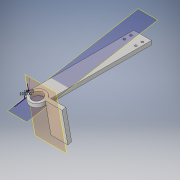
# Autodesk Inventor part: WheelIntakeMotorMount2.0
Saved by Autodesk Inventor 2017 (Build 210142000, 142)
## iProperties
Created: 2017-11-18
Part Number: WheelIntakeMotorMount2.0
Material: Generic
Document SubType Name: Modeling
Designer: User
Density: 1 g/cm^3
Appearance: Default
Author: User
Autodesk Inventor part; units mm, degrees
ref_plane "YZ Plane" through (0, 0, 0) normal (1, 0, 0) x (0, 1, 0)
ref_plane "XZ Plane" through (0, 0, 0) normal (0, 1, 0) x (-1, 0, 0)
ref_plane "XY Plane" through (0, 0, 0) normal (0, 0, 1) x (1, 0, 0)
sketch "Sketch1" plane through (0, 0, 0) normal (1, 0, 0) x (0, 1, 0)
  line L0 (0, 0) -> (21.59, 0)
  line L1 (21.59, 0) -> (21.59, -127)
  line L2 (21.59, -127) -> (0, -127)
  line L3 (0, -127) -> (0, 0)
  dimension "d0" = 21.59
  dimension "d1" = 127
  constraints: 8 end point, 2 parallel, 1 horizontal, 1 perpendicular
  measures "d0" distance of L1.end L2.end
  measures "d1" distance of L0.end L1.end
extrude "Extrusion1" add sketch "Sketch1" along normal blind 4.7625
sketch "Sketch2" plane through (0, 21.59, 0) normal (0, 1, 0) x (1, 0, 0)
  line L0 (0, 0) -> (-3.2071, -18.1884)
  line L1 (0, 0) -> (18.469, 0) construction
  line L2 (0, 0) -> (13.0579, -2.3025)
  line L3 (0, 0) -> (13.2594, 0) construction
  dimension "d4" = 100
  dimension "d24" = 10
  constraints: 8 end point, 2 equal length, 2 horizontal
  measures "d4" angle of L0 L1
  measures "d24" angle of L2 L3
ref_plane "Work Plane1" through (0, 21.59, 0) normal (-0.9848078, 0, -0.1736482) x (-0.1736482, 0, 0.9848078)
sketch "Sketch3" plane through (0, 21.59, 0) normal (-0.9848078, 0, -0.1736482) x (-0.1736482, 0, 0.9848078)
  line L0 (-0.827, 0) -> (-0.827, -21.59) projected
  line L1 (-0.827, -21.59) -> (-125.8976, -21.59) projected
  line L2 (-125.8976, -21.59) -> (-125.8976, 0) projected
  line L3 (-125.8976, 0) -> (-0.827, 0) projected
  line L4 (0, -21.59) -> (0, 0) projected
  line L5 (0, -21.59) -> (-0.827, -21.59) projected
  line L6 (-0.827, 0) -> (-0.827, -21.59) projected
  line L7 (0, 0) -> (-0.827, 0) projected
  line L8 (0, -21.59) -> (0, 0) projected
  circle A0 centre (0, -10.795) radius 9.525
  dimension "d5" = 19.05
  dimension "d6" = 21.59
  dimension "d7" = 10.795
  constraints: 1 centre point, 1 midpoint
  measures "d5" diameter of A0
  measures "d6" distance of L4.start L4.end
  measures "d7" distance from line of L7 A0.centre
extrude "Extrusion2" add sketch "Sketch3" against normal blind 4.7625 contours A0 L4 L0 | L0 A0 | A0 L4
sketch "Sketch5" plane through (4.6901, 10.795, 0.827) normal (0.9848078, 0, 0.1736482) x (0.1736482, 0, -0.9848078)
  circle A0 centre (0, 0) radius 9.525 projected
  point P0 (0, -10.795)
hole "Hole2" at (4.6901, 10.795, 0.827) direction (-0.9848078, 0, -0.1736482) diameter 12.954 end through all
ref_plane "Work Plane3" through (0, 0, 0) normal (-0.1736482, 0, 0.9848078) x (0, 1, 0)
sketch "Sketch9" plane through (4.7625, 0, 0) normal (1, 0, 0) x (0, 0, -1)
  line L0 (0, 0) -> (127, 0) projected
  line L1 (127, 0) -> (127, 21.59) projected
  line L2 (127, 21.59) -> (0, 21.59) projected
  line L3 (0, 21.59) -> (0, 20.284) projected
  ellipse E0 centre (-0.8398, 10.795) end of major axis (8.8322, 10.795) minor radius 9.525 (0, 1.306) -> (0, 20.284) ccw projected
  circle A0 centre (115.825, 10.795) radius 8
  line L4 (111.825, 17.7232) -> (119.825, 17.7232)
  line L5 (119.825, 17.7232) -> (119.825, 3.8668)
  line L6 (119.825, 3.8668) -> (111.825, 3.8668)
  line L7 (111.825, 3.8668) -> (111.825, 17.7232)
  line L8 (0, 1.306) -> (0, 0) projected
  dimension "d34" = 16
  dimension "d35" = 8
  dimension "d36" = 4
  dimension "d37" = 21.59
  dimension "d38" = 10.795
  dimension "d39" = 11.175
  constraints: 8 end point, 2 parallel, 2 point on circle, 1 centre point, 1 horizontal, 1 perpendicular, 1 other
  measures "d34" diameter of A0
  measures "d35" distance of L5.end L6.end
  measures "d36" distance from line of L5 A0.centre
  measures "d37" distance of L0.end L1.end
  measures "d38" distance from line of L2 A0.centre
  measures "d39" distance from line of L1 A0.centre
hole "Hole3" at (4.7625, 17.7232, -111.825) at (4.7625, 17.7232, -119.825) at (4.7625, 3.8668, -119.825) at (4.7625, 3.8668, -111.825) direction (-1, 0, 0) diameter 2.794 end through all
sketch "Sketch10" plane through (0, 0, 0) normal (-0.1736482, 0, 0.9848078) x (0, 1, 0)
  ellipse E0 centre (10.795, 0) end of major axis (10.795, -54.019) minor radius 9.525 (20.284, -4.6901) -> (1.27, 0) ccw projected
  line L0 (1.27, 0) -> (20.32, 0) projected
  ellipse E1 centre (10.795, 0) end of major axis (10.795, -54.019) minor radius 9.525 (20.32, 0) -> (1.306, -4.6901) ccw projected
  ellipse E2 centre (10.795, -4.836) end of major axis (1.27, -4.836) minor radius 1.6795 (20.284, -4.6901) -> (1.306, -4.6901) ccw projected
  line L1 (1.27, -4.7625) -> (20.32, -4.7625) projected
  ellipse E3 centre (3.8668, 20.8074) end of major axis (5.2638, 20.8074) minor radius 0.2426 projected
  ellipse E4 centre (17.7232, 19.4182) end of major axis (19.1202, 19.4182) minor radius 0.2426 projected
  ellipse E5 centre (17.7232, 20.8074) end of major axis (19.1202, 20.8074) minor radius 0.2426 projected
  ellipse E6 centre (3.8668, 19.4182) end of major axis (5.2638, 19.4182) minor radius 0.2426 projected
  ellipse E7 centre (10.795, 0) end of major axis (17.272, 0) minor radius 1.1421 (17.272, 0) -> (4.318, 0) ccw projected
  line L2 (17.272, 0) -> (20.32, 0) projected
  line L3 (20.32, 0) -> (21.59, 0) projected
  line L4 (21.59, 0) -> (21.59, 22.0533) projected
  line L5 (21.59, 22.0533) -> (0, 22.0533) projected
  line L6 (0, 22.0533) -> (0, 0) projected
  line L7 (0, 0) -> (1.27, 0) projected
  line L8 (1.27, 0) -> (4.318, 0) projected
  line L9 (20.32, 0) -> (1.27, 0) projected
  line L10 (3.0923, 0) -> (1.27, 0)
  line L11 (-19.1327, 0) -> (-19.1327, -4.7625)
  line L12 (-19.1327, -4.7625) -> (3.0923, -4.7625)
  line L13 (3.0923, -4.7625) -> (3.0923, 0)
  line L14 (-19.1327, -4.7625) -> (1.27, -4.7625)
  line L15 (1.27, 0) -> (1.27, 35.6235)
  line L16 (1.27, 35.6235) -> (-19.1327, 35.6235)
  line L17 (-19.1327, 35.6235) -> (-19.1327, -4.7625)
  dimension "d47" = 22.225
  dimension "d50" = 20.4027
  dimension "d53" = 4.7625
  dimension "d54" = 40.386
  constraints: 16 end point, 4 parallel, 2 horizontal, 2 perpendicular, 1 point on line, 8 other
  measures "d47" distance of L12.end L11.end
  measures "d50" distance of L15.end L16.end
  measures "d53" distance between parallel lines of L12 L10
  measures "d54" distance of L16.end L11.end
extrude "Extrusion4" add sketch "Sketch10" against normal blind 4.7625 contours L13 L1 L12 L11 L17 L16 L15 L5 L6 L7 E1 E2 | E2 E1 L0 L13 | L7 L6 L5 L15
equation "\"d7\" = 0.5 * d6"
equation "\"d36\" = 0.5 * d35"
equation "\"d38\" = 0.5 * d37"
body "Solid1"
